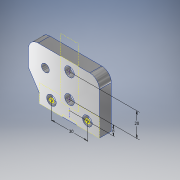
# Autodesk Inventor part: ZBaringBracket
Saved by Autodesk Inventor 2019 (Build 230136000, 136)
## iProperties
Created: 2018-10-14
Part Number: ZBaringBracket
Material: Aluminum 6061
Document SubType Name: Modeling
Designer: LillaHunden
Density: 2.7 g/cm^3
Appearance: Aluminum - Flat
Mass: 59.817 g
Surface Area: 75.5547 cm^2
Volume: 22.1545 cm^3
Author: LillaHunden
Autodesk Inventor part; units mm, degrees
ref_plane "YZ Plane" through (0, 0, 0) normal (1, 0, 0) x (0, 1, 0)
ref_plane "XZ Plane" through (0, 0, 0) normal (0, 1, 0) x (-1, 0, 0)
ref_plane "XY Plane" through (0, 0, 0) normal (0, 0, 1) x (1, 0, 0)
sketch "Sketch1" plane through (0, 0, 0) normal (0, 0, 1) x (1, 0, 0)
  line L0 (6, -5.5) -> (6, -7.5) construction
  line L1 (6, -7.5) -> (25, -7.5) construction
  line L2 (25, -7.5) -> (25, 7.5) construction
  line L3 (25, 7.5) -> (7.55, 7.5) construction
  line L4 (7.55, 7.5) -> (7.55, 2.5) construction
  line L5 (7.55, 2.5) -> (-7.55, 2.5) construction
  line L6 (-7.55, 2.5) -> (-7.55, 7.5) construction
  line L7 (-7.55, 7.5) -> (-25, 7.5) construction
  line L8 (-25, 7.5) -> (-25, -7.5) construction
  line L9 (-25, -7.5) -> (-6, -7.5) construction
  line L10 (-6, -7.5) -> (-6, -5.5) construction
  line L11 (-6, -5.5) -> (6, -5.5) construction
  line L12 (-7.45, 15.5) -> (7.55, 15.5) construction
  line L13 (-7.45, 2.5) -> (-7.45, 15.5) construction
  line L14 (7.55, 2.5) -> (-7.45, 2.5) construction
  line L15 (7.55, 2.5) -> (7.55, 15.5) construction
  line L16 (25, -7.5) -> (-34.185, -7.5)
  line L17 (-34.185, -7.5) -> (-34.185, 35.7282)
  line L18 (-34.185, 35.7282) -> (25, 35.7282)
  line L19 (25, 35.7282) -> (25, -7.5)
  circle A0 centre (15, 0) radius 1.621 projected
  circle A1 centre (-15, 0) radius 1.621 projected
  point P0 (0, 0)
  constraints: 8 end point, 2 parallel, 1 horizontal, 1 perpendicular, 1 point on line
extrude "Extrusion1" add sketch "Sketch1" along normal blind 10 contours L16 L17 L18 L19 | A0 | A1
sketch "Sketch4" plane through (0, 0, 10) normal (0, 0, 1) x (1, 0, 0)
  line L0 (6, -5.5) -> (6, -7.5) construction
  line L1 (6, -7.5) -> (25, -7.5) construction
  line L2 (25, -7.5) -> (25, 7.5) construction
  line L3 (25, 7.5) -> (7.55, 7.5) construction
  line L4 (7.55, 7.5) -> (7.55, 2.5) construction
  line L5 (7.55, 2.5) -> (-7.55, 2.5) construction
  line L6 (-7.55, 2.5) -> (-7.55, 7.5) construction
  line L7 (-7.55, 7.5) -> (-25, 7.5) construction
  line L8 (-25, 7.5) -> (-25, -7.5) construction
  line L9 (-25, -7.5) -> (-6, -7.5) construction
  line L10 (-6, -7.5) -> (-6, -5.5) construction
  line L11 (-6, -5.5) -> (6, -5.5) construction
  line L12 (0, 2.5) -> (0, -5.5) construction
  circle A0 centre (15, 0) radius 1.621 projected
  circle A1 centre (-15, 0) radius 1.621 projected
  point P0 (0, 0)
  point P1 (-15, 0)
  point P2 (15, 0)
  dimension "d8" = 30
  constraints: 2 end point, 2 midpoint, 1 symmetric about line
  measures "d8" distance of point (-15, 0) point (15, 0)
sketch "Sketch5" plane through (0, 0, 10) normal (0, 0, 1) x (1, 0, 0)
  point P0 (15, 0)
  point P1 (-15, 0)
hole "Hole1" at (15, 0, 10) at (-15, 0, 10) direction (0, 0, -1) diameter 4.3 depth 10 counterbore diameter 8 counterbore depth 4.5
sketch "Sketch6" plane through (0, 0, 10) normal (0, 0, 1) x (1, 0, 0)
  line L0 (7.55, 2.5) -> (7.55, 35.7282) construction
  line L1 (-7.45, 2.5) -> (-7.45, 35.7282) construction
  line L2 (-7.45, 52.1054) -> (7.55, 52.1054) construction
  line L3 (-7.45, 35.7282) -> (-7.45, 52.1054) construction
  line L4 (7.55, 35.7282) -> (-7.45, 35.7282) construction
  line L5 (7.55, 52.1054) -> (7.55, 35.7282) construction
  point P0 (0, 0)
  point P1 (0.0605, 28)
  point P2 (0.0605, 8)
  dimension "d16" = 20
  dimension "d17" = 8
  measures "d16" distance of point (0.06, 28) point (0.06, 8)
  measures "d17" vertical distance of point (0, 0) point (0.06, 8)
sketch "Sketch7" plane through (0, 0, 10) normal (0, 0, 1) x (1, 0, 0)
  point P0 (0.0605, 28)
  point P1 (0.0605, 8)
hole "Hole3" at (0.0605, 28, 10) at (0.0605, 8, 10) direction (0, 0, -1) diameter 4.3 depth 10 counterbore diameter 8 counterbore depth 4.5
sketch "Sketch8" plane through (0, 0, 10) normal (0, 0, 1) x (1, 0, 0)
  line L0 (-25, 7.5) -> (-25, -7.5) construction
  line L1 (-7.55, 7.5) -> (-25, 7.5) construction
  circle A0 centre (-20.1, 20.7) radius 5.5 construction
  line L2 (-34.185, -7.5) -> (-34.185, 35.7282) projected
  line L3 (-34.185, 14.1141) -> (-25, 0)
  line L4 (-25, -7.5) -> (-25, 0)
  line L5 (-34.185, 14.1141) -> (-34.185, 26.4425)
  line L6 (-34.185, 35.7282) -> (25, 35.7282) projected
  line L7 (-34.185, -7.5) -> (25, -7.5) projected
  point P0 (0, 0)
  constraints: 6 end point, 2 midpoint, 1 collinear, 1 point on line
extrude "Extrusion4" cut sketch "Sketch8" against normal through all
fillet "Fillet1" radius 3 1 edges at (-25, 0, 5)
fillet "Fillet2" radius 3 1 edges at (-34.185, 14.1141, 5)
fillet "Fillet4" radius 8 1 edges at (-34.185, 35.7282, 5)
fillet "Fillet5" radius 8 1 edges at (25, 35.7282, 5)
sketch "Sketch9" plane through (0, 0, 0) normal (0, 0, -1) x (-1, 0, 0)
  circle A0 centre (20.1, 20.7) radius 4.765
  arc A1 (21.2721, 23.6507) -> (18.4534, 23.4146) centre (20.1, 20.7) ccw projected
  point P0 (0, 0)
  dimension "d32" = 9.53
  constraints: 1 centre point
  measures "d32" diameter of A0
extrude "Extrusion5" cut sketch "Sketch9" against normal blind 3.3
sketch "Sketch10" plane through (-20.1, 20.7, 3.3) normal (0, 0, -1) x (-1, 0, 0)
  circle A0 centre (0, 0) radius 3.25
  point P0 (-20.1, -20.7)
  dimension "d35" = 6.5
  constraints: 1 centre point
  measures "d35" diameter of A0
extrude "Extrusion6" cut sketch "Sketch10" against normal through all
body "Solid1"
